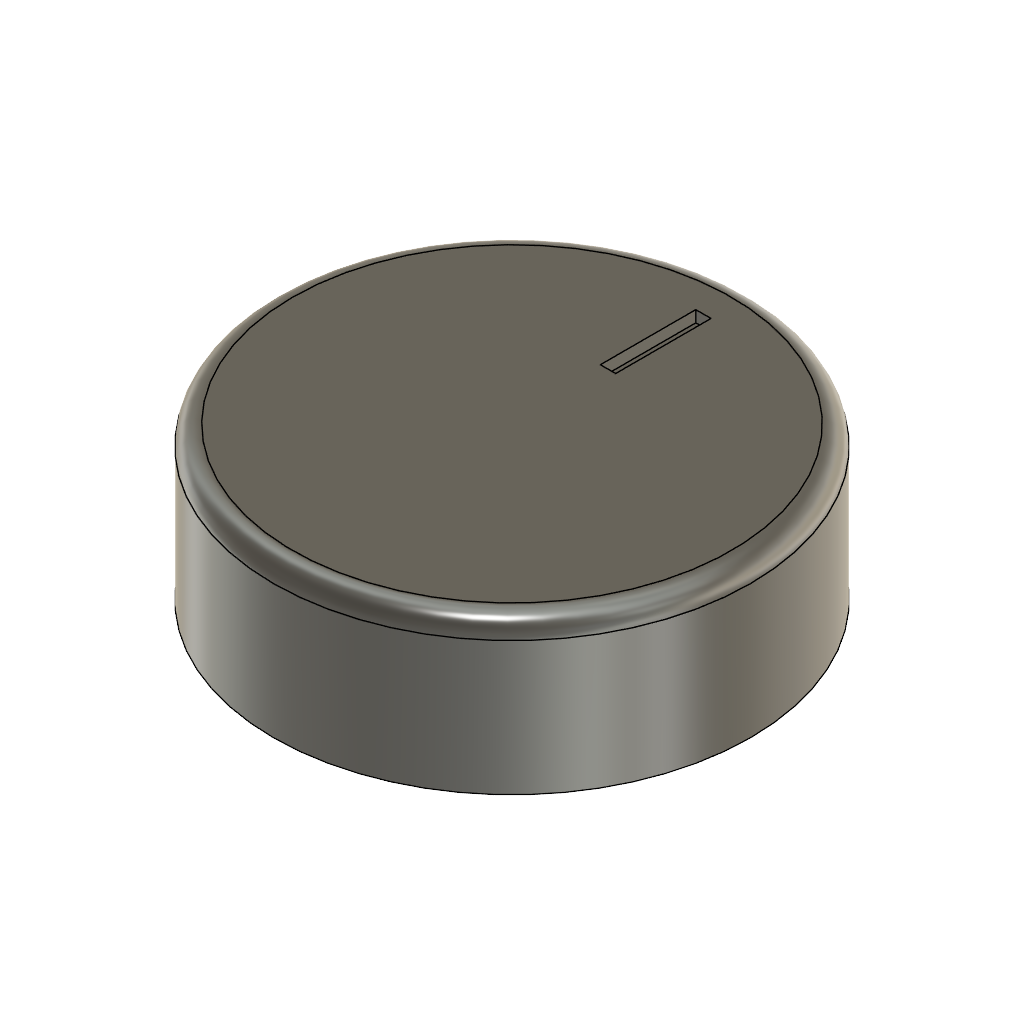
bouton-molette (Autodesk Fusion 360 design; units mm, degrees)
part number: 2026-10-03-17-31-33-729
Autodesk Fusion 360 part; units mm, degrees
sketch "Esquisse1" plane through (0, 0, 0) normal (0, 0, 1) x (1, 0, 0)
  circle A0 centre (0, 0) radius 12.5
  dimension "d9" = 25
  constraint coincident A0.centre origin
  measures "d9" diameter of A0
extrude "Extrusion1" add sketch "Esquisse1" along normal blind 8
fillet "Congé1" radius 1 1 edges at (-11.6541, -4.5202, 8)
sketch "Esquisse2" plane through (0, 0, 0) normal (0, 0, -1) x (1, 0, 0)
  circle A0 centre (0, 0) radius 12.5
  circle A1 centre (0, 0) radius 3.1
  line L0 (1.6, 2.6552) -> (1.6, -2.6552)
  dimension "d14" = 6.2
  dimension "d16" = 1.6
  constraint coincident A0.centre A1.centre
  constraint coincident A1 L0.start
  constraint coincident A1 L0.end
  constraint vertical L0
  measures "d14" diameter of A1
  measures "d16" distance of A0.centre L0
extrude "Extrusion2" cut sketch "Esquisse2" against normal blind 6 contours A1 L0 picked at (-0.3276, -0.4827)
sketch "Esquisse3" plane through (0, 0, 8) normal (0, 0, 1) x (-1, 0, 0)
  circle A0 centre (0, 0) radius 11.5
  line L0 (-0.431, -5) -> (0.369, -5)
  line L1 (0.369, -5) -> (0.369, -10)
  line L2 (0.369, -10) -> (-0.431, -10)
  line L3 (-0.431, -10) -> (-0.431, -5)
  line L4 (-0.431, -5) -> (0.369, -10) construction
  line L5 (0.369, -5) -> (-0.431, -10) construction
  point P0 (-0.031, -7.5)
  dimension "d19" = 5
  dimension "d20" = 0.8
  constraint horizontal L0
  constraint perpendicular L0 L1
  constraint parallel L0 L2
  constraint parallel L1 L3
  constraint coincident L4 P0
  constraint coincident L5 P0
  measures "d19" distance of L0.end L1.end
  measures "d20" distance of L1.end L2.end
extrude "Extrusion3" cut sketch "Esquisse3" against normal blind 0.6 contours L0 L1 L2 L3
sketch "Esquisse4" plane through (0, 0, 0) normal (0, 0, -1) x (1, 0, 0)
  line L0 (1.6, 2.6552) -> (1.6, -2.6552)
  arc A0 (1.6, 2.6552) -> (1.6, -2.6552) centre (0, 0) ccw
  circle A1 centre (0, 0) radius 12.5
  circle A2 centre (-10, 0) radius 0.4
  dimension "d23" = 0.8
  measures "d23" diameter of A2
extrude "Extrusion4" cut sketch "Esquisse4" against normal blind 0.8 contours A2
pattern_linear "Réseau R1" count 2 spacing 1.5 along (1, 0, 0) of "Extrusion4"
equation "d_bouton = 25 mm"
equation "h_bouton = 8 mm"
equation "r_conge = 1 mm"
equation "d_axe = 6 mm"
equation "e_meplat = 4.5 mm"
equation "l_meplat = 7 mm"
equation "p_alesage = 6 mm"
equation "jeu_axe = 0.2 mm"
equation "d9 = d_bouton"
equation "d10 = h_bouton"
equation "d13 = r_conge"
equation "d14 = d_axe + jeu_axe"
equation "d16 = ( e_meplat + jeu_axe ) - ( d_axe + jeu_axe ) / 2"
equation "d17 = -p_alesage"
